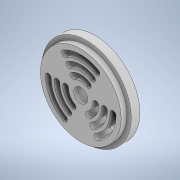
# Autodesk Inventor part: Мое седло
Saved by Autodesk Inventor 2021 (Build 250183000, 183)
## iProperties
Created: 2020-11-07
Part Number: Мое седло
Material: Типовые
Document SubType Name: Modeling
Designer: Тимоха
Density: 1 g/cm^3
Appearance: По умолчанию
Author: Тимоха
Autodesk Inventor part; units mm, degrees
ref_plane "YZ Plane" through (0, 0, 0) normal (1, 0, 0) x (0, 1, 0)
ref_plane "XZ Plane" through (0, 0, 0) normal (0, 1, 0) x (-1, 0, 0)
ref_plane "XY Plane" through (0, 0, 0) normal (0, 0, 1) x (1, 0, 0)
sketch "Эскиз1" plane through (0, 0, 0) normal (0, 0, 1) x (1, 0, 0)
  circle A0 centre (0, 0) radius 77.5
  dimension "d0" = 155
  constraints: 1 centre point, 1 coincident
  measures "d0" diameter of A0
extrude "Выдавливание1" add sketch "Эскиз1" along normal blind 15
sketch "Эскиз2" plane through (0, 0, 15) normal (0, 0, 1) x (1, 0, 0)
  circle A0 centre (0, 0) radius 70
  dimension "d3" = 140
  constraints: 1 centre point, 1 coincident
  measures "d3" diameter of A0
extrude "Выдавливание2" add sketch "Эскиз2" along normal blind 10
sketch "Эскиз3" plane through (0, 0, 0) normal (0, 0, -1) x (-1, 0, 0)
  circle A0 centre (0, 0) radius 70
  dimension "d6" = 140
  constraints: 1 centre point, 1 coincident
  measures "d6" diameter of A0
extrude "Выдавливание3" add sketch "Эскиз3" along normal blind 5
sketch "Эскиз5" plane through (0, 0, -5) normal (0, 0, -1) x (-1, 0, 0)
  circle A0 centre (0, 0) radius 65
  dimension "d9" = 130
  constraints: 1 centre point, 1 coincident
  measures "d9" diameter of A0
extrude "Выдавливание4" add sketch "Эскиз5" along normal blind 2
sketch "Эскиз6" plane through (0, 0, 25) normal (0, 0, 1) x (1, 0, 0)
  circle A0 centre (0, 0) radius 12
  dimension "d12" = 24
  constraints: 1 centre point, 1 coincident
  measures "d12" diameter of A0
extrude "Выдавливание5" cut sketch "Эскиз6" against normal through all
sketch "Эскиз7" plane through (0, 0, -7) normal (0, 0, -1) x (-1, 0, 0)
  arc A0 (11.25, 19.4856) -> (-11.25, 19.4856) centre (0, 0) ccw
  arc A1 (15, 25.9808) -> (-15, 25.9808) centre (0, 0) ccw
  arc A2 (18.75, 32.476) -> (-18.75, 32.476) centre (0, 0) ccw
  arc A3 (22.5, 38.9711) -> (-22.5, 38.9711) centre (0, 0) ccw
  arc A4 (26.25, 45.4663) -> (-26.25, 45.4663) centre (0, 0) ccw
  arc A5 (30, 51.9615) -> (-30, 51.9615) centre (0, 0) ccw
  line L0 (-29.5926, 0) -> (28.8589, 0)
  line L1 (28.8589, 0) -> (0, 0)
  arc A6 (11.25, 19.4856) -> (15, 25.9808) centre (13.125, 22.7332) ccw
  arc A7 (18.75, 32.476) -> (22.5, 38.9711) centre (20.625, 35.7235) ccw
  arc A8 (26.25, 45.4663) -> (30, 51.9615) centre (28.125, 48.7139) ccw
  line L2 (0, -108.5) -> (0, 108.5) projected
  arc A9 (-15, 25.9808) -> (-11.25, 19.4856) centre (-13.125, 22.7332) ccw
  arc A10 (-22.5, 38.9711) -> (-18.75, 32.476) centre (-20.625, 35.7235) ccw
  arc A11 (-30, 51.9615) -> (-26.25, 45.4663) centre (-28.125, 48.7139) ccw
  dimension "d15" = 45
  dimension "d16" = 60
  dimension "d17" = 75
  dimension "d18" = 90
  dimension "d19" = 105
  dimension "d20" = 120
  constraints: 24 point on circle, 12 centre point, 9 symmetric about line, 6 coincident, 4 end point, 1 collinear, 1 horizontal, 3 other
  measures "d15" diameter of A0
  measures "d16" diameter of A1
  measures "d17" diameter of A2
  measures "d18" diameter of A3
  measures "d19" diameter of A4
  measures "d20" diameter of A5
extrude "Выдавливание6" cut sketch "Эскиз7" against normal blind 5
sketch "Эскиз8" plane through (0, 0, 25) normal (0, 0, 1) x (1, 0, 0)
  arc A0 (10.625, 18.403) -> (-10.625, 18.403) centre (0, 0) ccw
  arc A1 (18.125, 31.3934) -> (-18.125, 31.3934) centre (0, 0) ccw
  arc A2 (18.75, 32.476) -> (-18.75, 32.476) centre (0, 0) ccw projected
  arc A3 (23.125, 40.0537) -> (-23.125, 40.0537) centre (0, 0) ccw
  arc A4 (25.625, 44.3838) -> (-25.625, 44.3838) centre (0, 0) ccw
  arc A5 (30.625, 53.0441) -> (-30.625, 53.0441) centre (0, 0) ccw
  line L0 (37.1026, 0) -> (0, 0)
  arc A6 (18.125, 31.3934) -> (23.125, 40.0537) centre (20.625, 35.7235) ccw
  arc A7 (10.625, 18.403) -> (15.625, 27.0633) centre (13.125, 22.7332) ccw
  arc A8 (25.625, 44.3838) -> (30.625, 53.0441) centre (28.125, 48.7139) ccw
  line L1 (0, -108.5) -> (0, 108.5) projected
  arc A9 (-23.125, 40.0537) -> (-18.125, 31.3934) centre (-20.625, 35.7235) ccw
  arc A10 (-15.625, 27.0633) -> (-10.625, 18.403) centre (-13.125, 22.7332) ccw
  arc A11 (-30.625, 53.0441) -> (-25.625, 44.3838) centre (-28.125, 48.7139) ccw
  arc A12 (15.625, 27.0633) -> (-15.625, 27.0633) centre (0, 0) ccw
  dimension "d31" = 42.5
  dimension "d33" = 72.5
  dimension "d34" = 92.5
  dimension "d35" = 102.5
  dimension "d36" = 122.5
  constraints: 24 point on circle, 12 centre point, 9 symmetric about line, 5 coincident, 2 end point, 1 horizontal, 3 other
  measures "d31" diameter of A0
  measures "d33" diameter of A1
  measures "d34" diameter of A3
  measures "d35" diameter of A4
  measures "d36" diameter of A5
sketch "Эскиз9" plane through (0, 0, -2) normal (0, 0, -1) x (-1, 0, 0)
  arc A0 (30, 51.9615) -> (-30, 51.9615) centre (0, 0) ccw projected
  arc A1 (-30, 51.9615) -> (-26.25, 45.4663) centre (-28.125, 48.7139) ccw projected
  arc A2 (26.25, 45.4663) -> (-26.25, 45.4663) centre (0, 0) ccw projected
  arc A3 (26.25, 45.4663) -> (30, 51.9615) centre (28.125, 48.7139) ccw projected
  arc A4 (22.5, 38.9711) -> (-22.5, 38.9711) centre (0, 0) ccw projected
  arc A5 (-22.5, 38.9711) -> (-18.75, 32.476) centre (-20.625, 35.7235) ccw projected
  arc A6 (18.75, 32.476) -> (-18.75, 32.476) centre (0, 0) ccw projected
  arc A7 (18.75, 32.476) -> (22.5, 38.9711) centre (20.625, 35.7235) ccw projected
  arc A8 (11.25, 19.4856) -> (-11.25, 19.4856) centre (0, 0) ccw projected
  arc A9 (11.25, 19.4856) -> (15, 25.9808) centre (13.125, 22.7332) ccw projected
  arc A10 (15, 25.9808) -> (-15, 25.9808) centre (0, 0) ccw projected
  arc A11 (-15, 25.9808) -> (-11.25, 19.4856) centre (-13.125, 22.7332) ccw projected
loft "Лофт1" cut profiles "Эскиз8" section 1 edges at (0, 60, -2) (31.3726, 46.8389, -2) (0, 52.5, -2) (-31.3726, 46.8389, -2) contours A4 L1 A5 A8 | A4 A11 A5 L1
loft "Лофт2" cut profiles "Эскиз8" section 2 edges at (0, 45, -2) (23.8726, 33.8485, -2) (0, 37.5, -2) (-23.8726, 33.8485, -2) contours A1 L1 A3 A6 | A1 A9 A3 L1
loft "Лофт3" cut profiles "Эскиз8" section 1 edges at (0, 22.5, -2) (-16.3726, 20.8582, -2) (0, 30, -2) (16.3726, 20.8582, -2) contours A0 L1 A12 A7 | A0 A10 A12 L1
pattern_circular "Круговой массив1" count 3 over 360 about axis through (0, 0, -10) along (0, 0, 1) of "Лофт1", "Лофт2", "Лофт3", "Выдавливание6"
